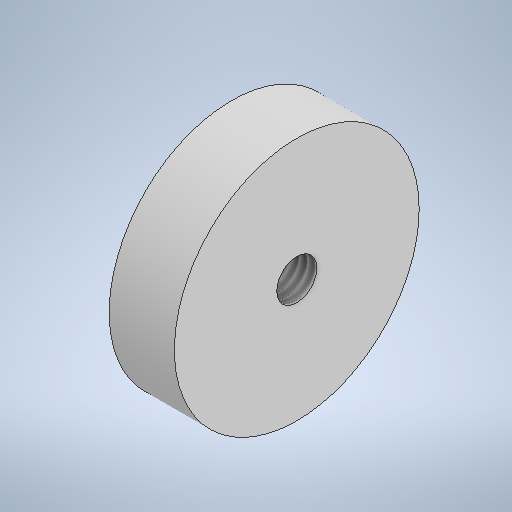
# Autodesk Inventor part: 20
Saved by Autodesk Inventor 2025.1 (Build 291241000, 241)
## iProperties
Created: 2024-09-18
Part Number: 20
Material: Generisch
Document SubType Name: Modeling
Designer: ffogue
Density: 1 g/cm^3
Appearance: Vorgabe
Author: ffogue
Autodesk Inventor part; units mm, degrees
ref_plane "YZ Plane" through (0, 0, 0) normal (1, 0, 0) x (0, 1, 0)
ref_plane "XZ Plane" through (0, 0, 0) normal (0, 1, 0) x (-1, 0, 0)
ref_plane "XY Plane" through (0, 0, 0) normal (0, 0, 1) x (1, 0, 0)
sketch "Sketch1" plane through (0, 0, 0) normal (0, 0, 1) x (1, 0, 0)
  line L0 (0, 0) -> (0, 2.4495)
  line L1 (0, 2.4495) -> (1, 7.5)
  line L2 (1, 7.5) -> (5, 7.5)
  line L3 (5, 7.5) -> (5, 0)
  line L4 (5, 0) -> (0, 0)
  point P0 (3, 7.5)
  point P1 (2.5, 0)
  dimension "d0" = 15
  dimension "d1" = 7
  dimension "d2" = 4
  dimension "d3" = 5
  constraints: 10 end point, 3 perpendicular, 2 midpoint, 1 vertical
  measures "d0" diameter of point (3, 7.5) L4
  measures "d1" diameter of L0.end point (2.5, 0)
  measures "d2" distance of L1.end L2.end
  measures "d3" distance between parallel lines of L3 L0
revolve "Revolution1" add sketch "Sketch1" angle 360 about axis through (5, 0, 0) along (-1, 0, 0)
sketch "Sketch2" plane through (5, 0, 0) normal (1, 0, 0) x (0, 0, -1)
  circle A0 centre (0, 0) radius 7.5 projected
  point P0 (0, 0)
  constraints: 1 coincident
hole "Hole1" at (5, 0, 0) direction (-1, 0, 0) diameter 2.459 depth 5 thread size "M3x0.5" class "6H" standard "ISO Metric profile"
body "Solid1"
